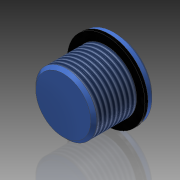
# Autodesk Inventor part: Flutschraube
Saved by Autodesk Inventor 2015 SP2 (Build 190223200, 223)
## iProperties
Created: 2016-11-08
Part Number: Flutschraube
Material: Allgemein
Document SubType Name: Modeling
Designer: Gruber
Density: 1 g/cm^3
Appearance: Glatt - schwarz
RuleStatus: InUse
AfterDocSave0: file://Projektnummer
Author: Gruber
And.-Index: 0
Autodesk Inventor part; units mm, degrees
ref_plane "YZ Plane" through (0, 0, 0) normal (1, 0, 0) x (0, 1, 0)
ref_plane "XZ Plane" through (0, 0, 0) normal (0, 1, 0) x (-1, 0, 0)
ref_plane "XY Plane" through (0, 0, 0) normal (0, 0, 1) x (1, 0, 0)
sketch "Skizze1" plane through (0, 0, 0) normal (0, 0, 1) x (1, 0, 0)
  circle A0 centre (0, 0) radius 25
  dimension "d0" = 50
  constraints: 1 centre point, 1 coincident
  measures "d0" diameter of A0
extrude "Extrusion1" add sketch "Skizze1" along normal blind 5
sketch "Skizze2" plane through (0, 0, 5) normal (0, 0, 1) x (1, 0, 0)
  circle A0 centre (0, 0) radius 20
  dimension "d3" = 40
  constraints: 1 centre point, 1 coincident
  measures "d3" diameter of A0
extrude "Extrusion2" add sketch "Skizze2" along normal blind 30
thread "Gewinde1" size "M40x3" class "6g" standard "ISO Metric profile" full length
chamfer "Fase1" distance 2 angle 45 2 edges at (-20, 0, 35) (-25, 0, 0)
sketch "Skizze3" plane through (0, 0, 0) normal (0, 0, -1) x (-1, 0, 0)
  line L0 (-15, -4) -> (15, -4)
  line L1 (15, -4) -> (15, 4)
  line L2 (15, 4) -> (-15, 4)
  line L3 (-15, 4) -> (-15, -4)
  line L4 (-15, -4) -> (15, 4) construction
  line L5 (15, -4) -> (-15, 4) construction
  line L6 (-4, -15) -> (4, -15)
  line L7 (4, -15) -> (4, 15)
  line L8 (4, 15) -> (-4, 15)
  line L9 (-4, 15) -> (-4, -15)
  line L10 (-4, -15) -> (4, 15) construction
  line L11 (4, -15) -> (-4, 15) construction
  point P0 (0, 0)
  dimension "d11" = 30
  dimension "d12" = 30
  dimension "d13" = 8
  dimension "d14" = 8
  constraints: 24 end point, 4 midpoint, 4 parallel, 2 horizontal, 2 perpendicular
  measures "d11" distance of L6.end L7.end
  measures "d12" distance of L0.start L0.end
  measures "d13" distance of L0.end L1.end
  measures "d14" distance of L7.end L8.end
extrude "Extrusion3" cut sketch "Skizze3" against normal blind 8
fillet "Rundung1" radius 2 12 edges at (-4, 9.5, 0) (0, 15, 0) (4, 9.5, 0) (9.5, 4, 0) (15, 0, 0) (9.5, -4, 0) (4, -9.5, 0) (-4, -9.5, 0) (0, -15, 0) (-9.5, -4, 0) (-15, 0, 0) (-9.5, 4, 0)
sketch "Skizze4" plane through (0, 0, 5) normal (0, 0, 1) x (1, 0, 0)
  circle A0 centre (0, 0) radius 25.5
  dimension "d18" = 51
  constraints: 1 centre point, 1 coincident
  measures "d18" diameter of A0
extrude "Extrusion4" add sketch "Skizze4" along normal blind 2
